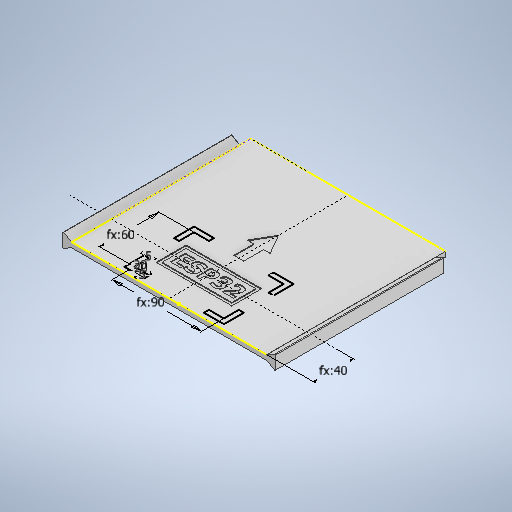
# Autodesk Inventor part: Suelo2
Saved by Autodesk Inventor 2025.1 (Build 291241000, 241)
## iProperties
Created: 2025-11-20
Part Number: Suelo2
Material: Genérico
Document SubType Name: Modeling
Designer: Diego
Density: 1 g/cm^3
Appearance: Valor por defecto
Author: Diego
Autodesk Inventor part; units mm, degrees
ref_plane "YZ Plane" through (0, 0, 0) normal (1, 0, 0) x (0, 1, 0)
ref_plane "XZ Plane" through (0, 0, 0) normal (0, 1, 0) x (-1, 0, 0)
ref_plane "XY Plane" through (0, 0, 0) normal (0, 0, 1) x (1, 0, 0)
sketch "Boceto1" plane through (0, 0, 0) normal (0, 0, 1) x (1, 0, 0)
  line L0 (-107.4375, 9.96) -> (-116.4375, 15.1562)
  line L1 (-116.4375, 15.1562) -> (-116.4375, -0.2361)
  line L2 (-116.4375, -0.2361) -> (-107.4375, 4.96)
  line L3 (-107.4375, 9.96) -> (-98.4042, 9.96) construction
  line L4 (-107.4375, 4.96) -> (-97.9616, 4.96) construction
  line L5 (-107.4375, 12.46) -> (-107.4375, 9.96) construction
  line L6 (-107.4375, 12.46) -> (-107.4375, 9.96) construction
  line L7 (-107.4375, 2.46) -> (-107.4375, 4.96) construction
  line L8 (88.5625, 12.46) -> (88.5625, 9.96) construction
  line L9 (88.5625, 12.46) -> (88.5625, 9.96) construction
  line L10 (97.5625, -0.2361) -> (88.5625, 4.96)
  line L11 (88.5625, 9.96) -> (97.5625, 15.1562)
  line L12 (97.5625, 15.1562) -> (97.5625, -0.2361)
  line L13 (88.5625, 4.96) -> (88.5625, 4.96) construction
  line L14 (88.5625, 4.96) -> (88.5625, 4.96) construction
  line L15 (88.5625, 4.96) -> (88.5625, 4.96)
  line L16 (88.5625, 7.46) -> (88.5625, 4.96)
  line L17 (88.5625, 4.96) -> (88.5625, 4.96)
  line L18 (88.5625, 9.96) -> (88.5625, 7.46)
  line L19 (-107.4375, 9.96) -> (-107.4375, 4.96)
  point P0 (0, 0)
  point P1 (-116.4375, 7.46)
  point P2 (97.5625, 7.46)
  point P3 (93.0625, 12.5581)
  point P4 (-111.9375, 12.5581)
  dimension "d0" = 60
  constraints: 40 end point, 5 vertical, 3 midpoint, 2 horizontal, 1 collinear, 1 parallel, 5 other
  measures "d0" angle of L0 L1
extrude "Extrusión1" add sketch "Boceto1" against normal blind 170
sketch "Boceto2" plane through (0, 0, 0) normal (0, 0, 1) x (1, 0, 0)
  line L0 (-107.4375, 9.96) -> (-107.4375, 4.96) projected
  line L1 (97.5625, -0.2361) -> (88.5625, 4.96) projected
  line L2 (-107.4375, 9.96) -> (88.5625, 9.96)
  line L3 (88.5625, 9.96) -> (88.5625, 4.96)
  line L4 (88.5625, 4.96) -> (-107.4375, 4.96)
  line L5 (-107.4375, 4.96) -> (-107.4375, 9.96)
  point P0 (0, 0)
  constraints: 8 end point, 2 parallel, 1 horizontal, 1 perpendicular
extrude "Extrusión2" add sketch "Boceto2" against normal blind 180
sketch "Boceto3" plane through (-107.4375, 9.96, 0) normal (0, 1, 0) x (1, 0, 0)
  line L0 (0, 0) -> (196, 0) projected
  line L1 (0, 0) -> (0, 170) projected
  line L2 (0, 180) -> (64.5, 180) construction
  line L3 (0, 42.5) -> (0, 180) construction
  line L4 (0, 180) -> (196, 180) projected
  line L5 (0, 170) -> (0, 180) projected
  line L6 (196, 180) -> (0, 180) construction
  line L7 (98, 180) -> (98, 0) construction
  line L8 (53, 10) -> (68, 10)
  line L9 (68, 10) -> (68, 5)
  line L10 (68, 5) -> (48, 5)
  line L11 (48, 5) -> (48, 25)
  line L12 (48, 25) -> (53, 25)
  line L13 (53, 25) -> (53, 10)
  line L14 (-40.9224, 40) -> (227.6994, 40) construction
  line L15 (143, 10) -> (128, 10)
  line L16 (128, 10) -> (128, 5)
  line L17 (128, 5) -> (148, 5)
  line L18 (148, 5) -> (148, 25)
  line L19 (148, 25) -> (143, 25)
  line L20 (143, 25) -> (143, 10)
  line L21 (53, 70) -> (68, 70)
  line L22 (68, 70) -> (68, 75)
  line L23 (68, 75) -> (48, 75)
  line L24 (48, 75) -> (48, 55)
  line L25 (48, 55) -> (53, 55)
  line L26 (53, 55) -> (53, 70)
  line L27 (143, 70) -> (128, 70)
  line L28 (128, 70) -> (128, 75)
  line L29 (143, 55) -> (143, 70)
  line L30 (148, 55) -> (143, 55)
  line L31 (128, 75) -> (148, 75)
  line L32 (148, 75) -> (148, 55)
  point P0 (107.4375, 0)
  dimension "d22" = 5
  dimension "d23" = 20
  dimension "d24" = 5
  dimension "d26" = 20
  dimension "d55" = 90
  dimension "d56" = 60
  dimension "d57" = 40
  constraints: 56 end point, 18 symmetric about line, 4 horizontal, 3 perpendicular, 2 midpoint
  measures "d22" distance of L11.end L12.end
  measures "d23" distance of L10.end L11.end
  measures "d24" distance of L8.end L9.end
  measures "d26" distance of L9.end L10.end
  measures "d55" distance between parallel lines of L20 L13
  measures "d56" distance between parallel lines of L8 L21
  measures "d57" distance between parallel lines of L0 L14
sketch "Boceto4" plane through (-107.4375, 9.96, 0) normal (0, 1, 0) x (1, 0, 0)
  line L0 (98, 180) -> (98, 0) construction
  line L1 (131.5, 108) -> (196, 108) construction
  line L2 (131.5, 90) -> (196, 90) construction
  line L3 (131.5, 72) -> (196, 72) construction
  line L4 (163.75, 180) -> (163.75, 42.5) construction
  line L5 (131.5, 180) -> (143, 10) construction
  line L6 (93, 90) -> (93, 70)
  line L7 (93, 70) -> (103, 70)
  line L8 (103, 70) -> (103, 90)
  line L9 (103, 90) -> (93, 70) construction
  line L10 (93, 90) -> (103, 70) construction
  line L11 (93, 90) -> (86.453, 90)
  line L12 (86.453, 90) -> (98, 110)
  line L13 (98, 110) -> (109.547, 90)
  line L14 (109.547, 90) -> (103, 90)
  line L15 (196, 0) -> (0, 0) projected
  line L16 (60, 55) -> (136, 55) construction
  line L17 (136, 55) -> (136, 25) construction
  line L18 (136, 25) -> (60, 25) construction
  line L19 (60, 25) -> (60, 55) construction
  line L20 (60, 55) -> (136, 55)
  line L21 (136, 55) -> (136, 25)
  line L22 (136, 25) -> (60, 25)
  line L23 (60, 25) -> (60, 55)
  line L24 (133, 52) -> (63, 52)
  line L25 (63, 52) -> (63, 28)
  line L26 (63, 28) -> (133, 28)
  line L27 (133, 28) -> (133, 52)
  line L28 (-40.9224, 40) -> (227.6994, 40) construction
  line L29 (66.7601, 32.5) -> (66.7601, 47.5)
  line L30 (66.7601, 47.5) -> (76.8979, 47.5)
  line L31 (76.8979, 47.5) -> (76.8979, 44.6434)
  line L32 (76.8979, 44.6434) -> (70.5041, 44.6434)
  line L33 (70.5041, 44.6434) -> (70.5041, 42.0057)
  line L34 (70.5041, 42.0057) -> (76.3995, 42.0057)
  line L35 (76.3995, 42.0057) -> (76.3995, 39.1491)
  line L36 (76.3995, 39.1491) -> (70.5041, 39.1491)
  line L37 (70.5041, 39.1491) -> (70.5041, 35.3566)
  line L38 (70.5041, 35.3566) -> (76.8979, 35.3566)
  line L39 (76.8979, 35.3566) -> (76.8979, 32.5)
  line L40 (76.8979, 32.5) -> (66.7601, 32.5)
  spline S0 degree 2 poles (84.0818, 32.2326) (82.3558, 32.2326) (79.7545, 32.9011) (78.6361, 33.3874) knots 0 0 0 1 2 2 2
  line L41 (78.6361, 33.3874) -> (78.6361, 36.9611)
  line L42 (78.6361, 36.9611) -> (78.9765, 36.9611)
  spline S1 degree 2 poles (78.9765, 36.9611) (80.107, 36.0008) (82.8177, 34.9676) (84.094, 34.9676) knots 0 0 0 1 2 2 2
  spline S2 degree 2 poles (84.094, 34.9676) (84.4222, 34.9676) (85.4797, 35.1135) (85.7958, 35.2593) knots 0 0 0 1 2 2 2
  spline S3 degree 2 poles (85.7958, 35.2593) (86.1848, 35.4295) (86.7318, 36.0494) (86.7318, 36.5478) knots 0 0 0 1 2 2 2
  spline S4 degree 2 poles (86.7318, 36.5478) (86.7318, 37.1191) (85.8444, 37.8241) (85.2366, 37.9822) knots 0 0 0 1 2 2 2
  spline S5 degree 2 poles (85.2366, 37.9822) (84.4708, 38.1888) (82.7326, 38.5413) (81.9668, 38.8088) knots 0 0 0 1 2 2 2
  spline S6 degree 2 poles (81.9668, 38.8088) (80.2285, 39.4165) (78.7212, 41.4951) (78.7212, 43.0511) knots 0 0 0 1 2 2 2
  spline S7 degree 2 poles (78.7212, 43.0511) (78.7212, 45.154) (82.2828, 47.7674) (84.957, 47.7674) knots 0 0 0 1 2 2 2
  spline S8 degree 2 poles (84.957, 47.7674) (86.2942, 47.7674) (88.9441, 47.2204) (89.9895, 46.7585) knots 0 0 0 1 2 2 2
  line L43 (89.9895, 46.7585) -> (89.9895, 43.3306)
  line L44 (89.9895, 43.3306) -> (89.6613, 43.3306)
  spline S9 degree 2 poles (89.6613, 43.3306) (88.8225, 44.0478) (86.4157, 45.0324) (85.1515, 45.0324) knots 0 0 0 1 2 2 2
  spline S10 degree 2 poles (85.1515, 45.0324) (84.6532, 45.0324) (83.8752, 44.8865) (83.4376, 44.6921) knots 0 0 0 1 2 2 2
  spline S11 degree 2 poles (83.4376, 44.6921) (83.0851, 44.534) (82.5746, 43.9019) (82.5746, 43.513) knots 0 0 0 1 2 2 2
  spline S12 degree 2 poles (82.5746, 43.513) (82.5746, 42.9295) (83.389, 42.2609) (84.5559, 41.9935) knots 0 0 0 1 2 2 2
  spline S13 degree 2 poles (84.5559, 41.9935) (85.3096, 41.8233) (86.7075, 41.4951) (87.5097, 41.2156) knots 0 0 0 1 2 2 2
  spline S14 degree 2 poles (87.5097, 41.2156) (89.0656, 40.6442) (90.5851, 38.748) (90.5851, 37.1921) knots 0 0 0 1 2 2 2
  spline S15 degree 2 poles (90.5851, 37.1921) (90.5851, 34.9554) (87.0721, 32.2326) (84.0818, 32.2326) knots 0 0 0 1 2 2 2
  spline S16 degree 2 poles (104.0535, 42.7715) (104.0535, 41.7261) (103.3849, 39.8298) (102.765, 39.1977) knots 0 0 0 1 2 2 2
  spline S17 degree 2 poles (102.765, 39.1977) (102.3882, 38.7966) (101.4643, 38.1402) (100.9173, 37.9092) knots 0 0 0 1 2 2 2
  spline S18 degree 2 poles (100.9173, 37.9092) (100.3582, 37.6783) (99.0575, 37.4109) (98.2553, 37.4109) knots 0 0 0 1 2 2 2
  line L45 (98.2553, 37.4109) -> (96.2861, 37.4109)
  line L46 (96.2861, 37.4109) -> (96.2861, 32.5)
  line L47 (96.2861, 32.5) -> (92.5178, 32.5)
  line L48 (92.5178, 32.5) -> (92.5178, 47.5)
  line L49 (92.5178, 47.5) -> (98.3404, 47.5)
  spline S19 degree 2 poles (98.3404, 47.5) (99.6288, 47.5) (101.513, 47.0259) (102.2788, 46.5154) knots 0 0 0 1 2 2 2
  spline S20 degree 2 poles (102.2788, 46.5154) (103.1297, 45.9441) (104.0535, 44.0721) (104.0535, 42.7715) knots 0 0 0 1 2 2 2
  spline S21 degree 2 poles (100.188, 42.6742) (100.188, 43.3185) (99.5802, 44.2301) (99.1669, 44.4003) knots 0 0 0 1 2 2 2
  spline S22 degree 2 poles (99.1669, 44.4003) (98.6321, 44.6313) (97.6596, 44.7042) (96.8209, 44.7042) knots 0 0 0 1 2 2 2
  line L50 (96.8209, 44.7042) -> (96.2861, 44.7042)
  line L51 (96.2861, 44.7042) -> (96.2861, 40.2066)
  line L52 (96.2861, 40.2066) -> (96.5535, 40.2066)
  spline S23 degree 2 poles (96.5535, 40.2066) (97.0762, 40.2066) (98.0243, 40.231) (98.3768, 40.2917) knots 0 0 0 1 2 2 2
  spline S24 degree 2 poles (98.3768, 40.2917) (98.6807, 40.3404) (99.3493, 40.6321) (99.5316, 40.8144) knots 0 0 0 1 2 2 2
  spline S25 degree 2 poles (99.5316, 40.8144) (99.9206, 41.1791) (100.188, 41.9935) (100.188, 42.6742) knots 0 0 0 1 2 2 2
  spline S26 degree 2 poles (116.6831, 37.0462) (116.6831, 35.94) (115.8687, 34.1288) (115.0786, 33.4968) knots 0 0 0 1 2 2 2
  spline S27 degree 2 poles (115.0786, 33.4968) (114.2885, 32.8647) (112.137, 32.184) (110.5932, 32.184) knots 0 0 0 1 2 2 2
  spline S28 degree 2 poles (110.5932, 32.184) (108.8428, 32.184) (106.3387, 32.7674) (105.5486, 33.1321) knots 0 0 0 1 2 2 2
  line L53 (105.5486, 33.1321) -> (105.5486, 36.3898)
  line L54 (105.5486, 36.3898) -> (105.9133, 36.3898)
  spline S29 degree 2 poles (105.9133, 36.3898) (106.7399, 35.8671) (108.9643, 35.0891) (109.8882, 35.0891) knots 0 0 0 1 2 2 2
  spline S30 degree 2 poles (109.8882, 35.0891) (110.4352, 35.0891) (111.7115, 35.2836) (112.1491, 35.5997) knots 0 0 0 1 2 2 2
  spline S31 degree 2 poles (112.1491, 35.5997) (112.4895, 35.8549) (112.9028, 36.5964) (112.9028, 37.265) knots 0 0 0 1 2 2 2
  spline S32 degree 2 poles (112.9028, 37.265) (112.9028, 37.9335) (112.3193, 38.6507) (111.8331, 38.8209) knots 0 0 0 1 2 2 2
  spline S33 degree 2 poles (111.8331, 38.8209) (111.3468, 38.9911) (109.9976, 39.0276) (109.4749, 39.0276) knots 0 0 0 1 2 2 2
  line L55 (109.4749, 39.0276) -> (108.8306, 39.0276)
  line L56 (108.8306, 39.0276) -> (108.8306, 41.6653)
  line L57 (108.8306, 41.6653) -> (109.4263, 41.6653)
  spline S34 degree 2 poles (109.4263, 41.6653) (110.107, 41.6653) (111.2617, 41.7869) (111.6629, 41.9692) knots 0 0 0 1 2 2 2
  spline S35 degree 2 poles (111.6629, 41.9692) (112.064, 42.1637) (112.5138, 42.8444) (112.5138, 43.4279) knots 0 0 0 1 2 2 2
  spline S36 degree 2 poles (112.5138, 43.4279) (112.5138, 43.8898) (112.0883, 44.4611) (111.7844, 44.6191) knots 0 0 0 1 2 2 2
  spline S37 degree 2 poles (111.7844, 44.6191) (111.4198, 44.8015) (110.4473, 44.923) (110.107, 44.923) knots 0 0 0 1 2 2 2
  spline S38 degree 2 poles (110.107, 44.923) (109.56, 44.923) (108.4052, 44.6677) (107.8703, 44.4611) knots 0 0 0 1 2 2 2
  spline S39 degree 2 poles (107.8703, 44.4611) (107.4449, 44.3031) (106.5211, 43.7925) (106.3023, 43.6588) knots 0 0 0 1 2 2 2
  line L58 (106.3023, 43.6588) -> (105.9862, 43.6588)
  line L59 (105.9862, 43.6588) -> (105.9862, 46.8679)
  spline S40 degree 2 poles (105.9862, 46.8679) (106.7642, 47.1961) (109.3898, 47.816) (110.7634, 47.816) knots 0 0 0 1 2 2 2
  spline S41 degree 2 poles (110.7634, 47.816) (112.1005, 47.816) (114.0697, 47.3541) (114.7626, 46.9044) knots 0 0 0 1 2 2 2
  spline S42 degree 2 poles (114.7626, 46.9044) (115.5284, 46.4303) (116.2942, 44.9716) (116.2942, 44.06) knots 0 0 0 1 2 2 2
  spline S43 degree 2 poles (116.2942, 44.06) (116.2942, 42.7715) (114.8112, 40.8509) (113.5956, 40.5713) knots 0 0 0 1 2 2 2
  line L60 (113.5956, 40.5713) -> (113.5956, 40.4254)
  spline S44 degree 2 poles (113.5956, 40.4254) (114.1305, 40.3525) (115.1515, 39.9635) (115.6378, 39.5259) knots 0 0 0 1 2 2 2
  spline S45 degree 2 poles (115.6378, 39.5259) (116.0875, 39.137) (116.6831, 37.8971) (116.6831, 37.0462) knots 0 0 0 1 2 2 2
  line L61 (130.2002, 32.5) -> (119.175, 32.5)
  line L62 (119.175, 32.5) -> (119.175, 34.9433)
  spline S46 degree 2 poles (119.175, 34.9433) (120.5729, 36.0616) (122.8096, 38.0308) (123.6483, 38.9182) knots 0 0 0 1 2 2 2
  spline S47 degree 2 poles (123.6483, 38.9182) (124.7545, 40.0729) (125.7391, 41.8355) (125.7391, 42.7593) knots 0 0 0 1 2 2 2
  spline S48 degree 2 poles (125.7391, 42.7593) (125.7391, 43.8047) (124.487, 44.923) (123.3687, 44.923) knots 0 0 0 1 2 2 2
  spline S49 degree 2 poles (123.3687, 44.923) (122.7974, 44.923) (121.7763, 44.6434) (121.2536, 44.4246) knots 0 0 0 1 2 2 2
  spline S50 degree 2 poles (121.2536, 44.4246) (120.7431, 44.1937) (120.0138, 43.7075) (119.8314, 43.5859) knots 0 0 0 1 2 2 2
  line L63 (119.8314, 43.5859) -> (119.5397, 43.5859)
  line L64 (119.5397, 43.5859) -> (119.5397, 46.8558)
  spline S51 degree 2 poles (119.5397, 46.8558) (120.1718, 47.1596) (122.8703, 47.7917) (124.1224, 47.7917) knots 0 0 0 1 2 2 2
  spline S52 degree 2 poles (124.1224, 47.7917) (126.7966, 47.7917) (129.5438, 45.4092) (129.5438, 43.2577) knots 0 0 0 1 2 2 2
  spline S53 degree 2 poles (129.5438, 43.2577) (129.5438, 41.9327) (128.2917, 39.3801) (126.8452, 37.9214) knots 0 0 0 1 2 2 2
  spline S54 degree 2 poles (126.8452, 37.9214) (125.9335, 37.0219) (124.2196, 35.624) (123.8428, 35.3323) knots 0 0 0 1 2 2 2
  line L65 (123.8428, 35.3323) -> (130.2002, 35.3323)
  line L66 (130.2002, 35.3323) -> (130.2002, 32.5)
  point P0 (107.4375, 0)
  point P1 (64.5, 108)
  point P2 (0, 108)
  point P3 (64.5, 90)
  point P4 (0, 90)
  point P5 (64.5, 72)
  point P6 (0, 72)
  point P7 (64.5, 180)
  point P8 (53, 10)
  point P9 (32.25, 180)
  point P10 (32.25, 42.5)
  point P11 (98, 80)
  dimension "d30" = 10
  dimension "d31" = 20
  dimension "d33" = 60
  dimension "d34" = 60
  dimension "d35" = 60
  dimension "d37" = 20
  dimension "d38" = 90
  dimension "d59" = 3
  dimension "d60" = 30
  dimension "d61" = 70
  constraints: 44 end point, 10 symmetric about line, 6 equal length, 3 point on line, 2 horizontal, 2 midpoint, 2 perpendicular, 1 vertical, 7 other
  measures "d30" distance of L6.end L7.end
  measures "d31" distance of L7.end L8.end
  measures "d33" angle of L11 L12
  measures "d34" angle of L14 L13
  measures "d35" angle of L13 L12
  measures "d37" distance from line of L14 L12.end
  measures "d38" distance between parallel lines of L15 L11
  measures "d59" distance between parallel lines of L20 L24
  measures "d60" distance of L22.end L19.end
  measures "d61" distance of L26.start L26.end
thicken "Engrosado1" operation cut thickness 0.15 both sides no extend neighbours no toward (-1, 0, 0) faces at (97.5625, 4.8947, -56.6667) (94.5625, 13.4241, -113.3333) (91.5625, 3.228, -113.3333)
thicken "Engrosado2" operation cut thickness 0.15 both sides no extend neighbours no toward (-0.5, -0.8660254, 0) faces at (-110.4375, 11.6921, -113.3333) (-116.4375, 10.0254, -56.6667) (-113.4375, 1.4959, -113.3333)
sketch "Boceto5" plane through (0, 0, 0) normal (0, 0, 1) x (1, 0, 0)
  line L0 (-116.2875, 14.8964) -> (-116.2875, 0.0237) projected
  line L1 (-116.2875, 7.46) -> (97.4125, 7.46) construction
  line L2 (97.4125, 0.0237) -> (97.4125, 14.8964) projected
  line L3 (88.5625, 9.96) -> (-107.4375, 9.96) projected
  line L4 (88.6375, 9.8301) -> (88.5625, 9.96) projected
  line L5 (-107.5125, 5.09) -> (-107.4375, 4.96) projected
  line L6 (-107.4375, 4.96) -> (88.5625, 4.96) projected
  line L7 (88.5625, 4.96) -> (88.6375, 5.09) projected
  line L8 (88.6375, 5.09) -> (97.4125, 0.0237) projected
  line L9 (97.4125, 0.0237) -> (97.4125, 14.8964) projected
  line L10 (97.4125, 14.8964) -> (88.6375, 9.8301) projected
  line L11 (88.6375, 9.8301) -> (88.5625, 9.96) projected
  line L12 (88.5625, 9.96) -> (-107.4375, 9.96) projected
  line L13 (-107.4375, 9.96) -> (-107.5125, 9.8301) projected
  line L14 (-107.5125, 9.8301) -> (-116.2875, 14.8964) projected
  line L15 (-116.2875, 14.8964) -> (-116.2875, 0.0237) projected
  line L16 (-116.2875, 0.0237) -> (-107.5125, 5.09) projected
  line L17 (88.5625, 9.96) -> (88.6375, 9.8301)
  line L18 (88.6375, 9.8301) -> (88.5625, 9.7868)
  line L19 (88.5625, 9.7868) -> (88.5625, 9.96)
  line L20 (-9.4375, 28.9561) -> (-9.4375, -11.7767) construction
  line L21 (97.4125, 14.8964) -> (88.6375, 9.8301) projected
  line L22 (88.6375, 5.09) -> (88.5625, 4.96)
  line L23 (88.6375, 5.09) -> (88.5625, 4.96)
  line L24 (88.5625, 4.96) -> (88.6375, 5.09)
  line L25 (88.6375, 5.09) -> (88.5625, 5.1333)
  line L26 (88.5625, 5.1333) -> (88.5625, 4.96)
  line L27 (-107.5125, 9.8301) -> (-107.4375, 9.96)
  line L28 (-107.4375, 4.96) -> (-107.5125, 5.09)
  line L29 (-107.5125, 9.8301) -> (-107.4375, 9.96)
  line L30 (-107.4375, 9.96) -> (-107.5125, 9.8301)
  line L31 (-107.5125, 9.8301) -> (-107.4375, 9.7868)
  line L32 (-107.4375, 9.7868) -> (-107.4375, 9.96)
  line L33 (-107.5125, 5.09) -> (-107.4375, 4.96)
  line L34 (-107.4375, 5.1333) -> (-107.4375, 4.96)
  line L35 (-107.5125, 5.09) -> (-107.4375, 4.96)
  line L36 (-107.4375, 4.96) -> (-107.5125, 5.09)
  line L37 (-107.5125, 5.09) -> (-107.4375, 5.1333)
  point P0 (0, 0)
  point P1 (-9.4375, 7.46)
  constraints: 42 end point, 19 symmetric about line, 3 midpoint, 2 vertical, 1 collinear, 1 point on line
extrude "Extrusión4" cut sketch "Boceto5" against normal through all contours L13 L32 L31 | L37 L34 L5 | L4 L18 L19 | L26 L25 L7
chamfer "Chaflán1" distance 1 angle 45 3 edges at (92.9875, 12.3416, -170) (97.4125, 7.46, -170) (92.9875, 2.5785, -170)
chamfer "Chaflán2" distance 1 angle 45 3 edges at (-111.8625, 12.3416, -170) (-116.2875, 7.46, -170) (-111.8625, 2.5785, -170)
fillet "Empalme1" radius 0.5 4 edges at (-116.2875, 14.8964, -84.5) (-116.2875, 0.0237, -84.5) (97.4125, 14.8964, -84.5) (97.4125, 0.0237, -84.5)
extrude "Extrusión5" cut sketch "Boceto4" against normal blind 0.8
equation "\"d3\" = L_base"
equation "\"L_base\" = 180"
equation "\"W_Pi\" = 64.5"
equation "\"L_Pi\" = 95"
equation "\"Font\" = 36"
